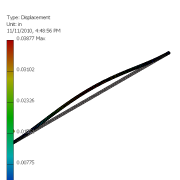
# Autodesk Inventor part: Aluminum Extrusion
Saved by Autodesk Inventor 2011 (Build 150239000, 239)
## iProperties
Created: 2010-11-11
Part Number: Aluminum Extrusion
Document SubType Name: Modeling
Designer: dfranz
Density: 2.71 g/cm^3
Material: Aluminum-6061
Mass: 2596.26 g
Surface Area: 10719.4 cm^2
Volume: 958.031 cm^3
Author: dfranz
Autodesk Inventor part; units mm, degrees
ref_plane "YZ Plane" through (0, 0, 0) normal (1, 0, 0) x (0, 1, 0)
ref_plane "XZ Plane" through (0, 0, 0) normal (0, 1, 0) x (-1, 0, 0)
ref_plane "XY Plane" through (0, 0, 0) normal (0, 0, 1) x (1, 0, 0)
sketch "Sketch1" plane through (0, 0, 0) normal (0, 0, 1) x (1, 0, 0)
  line L0 (-20.9356, 21.1258) -> (-11.0931, 21.1258)
  line L1 (8.9094, 1.1233) -> (8.9094, -8.7192)
  line L2 (-11.0931, -9.3542) -> (-20.9356, -9.3542)
  line L3 (-21.5706, 10.6483) -> (-21.5706, 20.4908)
  line L4 (-12.3631, 11.9183) -> (-0.2981, 11.9183)
  line L5 (-0.2981, 11.9183) -> (-0.2981, -0.1467)
  line L6 (-0.2981, -0.1467) -> (-12.3631, -0.1467)
  line L7 (-12.3631, -0.1467) -> (-12.3631, 11.9183)
  line L8 (-11.0931, 18.9668) -> (-19.4116, 18.9668)
  line L9 (-19.4116, 18.9668) -> (-19.4116, 10.6483)
  line L10 (-19.4116, -7.1952) -> (-11.0931, -7.1952)
  line L11 (6.7504, -7.1952) -> (6.7504, 1.1233)
  line L12 (-20.0466, 10.0133) -> (-20.9356, 10.0133)
  line L13 (-20.0466, 1.7583) -> (-20.9356, 1.7583)
  line L14 (-10.4581, 19.6018) -> (-10.4581, 20.4908)
  line L15 (-2.2031, 19.6018) -> (-2.2031, 20.4908)
  line L16 (7.3854, 10.0133) -> (8.2744, 10.0133)
  line L17 (7.3854, 1.7583) -> (8.2744, 1.7583)
  line L18 (-2.2031, -7.8302) -> (-2.2031, -8.7192)
  line L19 (-10.4581, -7.8302) -> (-10.4581, -8.7192)
  line L20 (-19.4116, 18.9668) -> (-16.2366, 18.9668)
  line L21 (-16.2366, 18.9668) -> (-16.2366, 16.4268)
  line L22 (-16.8716, 15.7918) -> (-19.4116, 15.7918)
  line L23 (-19.4116, 15.7918) -> (-19.4116, 18.9668)
  line L24 (3.5754, 18.9668) -> (6.7504, 18.9668)
  line L25 (6.7504, 18.9668) -> (6.7504, 15.7918)
  line L26 (6.7504, 15.7918) -> (4.2104, 15.7918)
  line L27 (3.5754, 16.4268) -> (3.5754, 18.9668)
  line L28 (6.7504, -7.1952) -> (3.5754, -7.1952)
  line L29 (3.5754, -7.1952) -> (3.5754, -4.6552)
  line L30 (4.2104, -4.0202) -> (6.7504, -4.0202)
  line L31 (6.7504, -4.0202) -> (6.7504, -7.1952)
  line L32 (-19.4116, -7.1952) -> (-16.2366, -7.1952)
  line L33 (-16.2366, -7.1952) -> (-16.2366, -4.0202)
  line L34 (-16.2366, -4.0202) -> (-19.4116, -4.0202)
  line L35 (-19.4116, -4.0202) -> (-19.4116, -7.1952)
  line L36 (-20.1736, 20.3638) -> (-17.6336, 20.3638)
  line L37 (-16.9986, 19.7288) -> (-16.9986, 17.1888)
  line L38 (-17.6336, 16.5538) -> (-20.1736, 16.5538)
  line L39 (-20.8086, 17.1888) -> (-20.8086, 19.7288)
  line L40 (7.5124, -8.5922) -> (4.9724, -8.5922)
  line L41 (4.3374, -7.9572) -> (4.3374, -5.4172)
  line L42 (4.9724, -4.7822) -> (7.5124, -4.7822)
  line L43 (8.1474, -5.4172) -> (8.1474, -7.9572)
  line L44 (7.5124, 20.3638) -> (4.9724, 20.3638)
  line L45 (4.3374, 19.7288) -> (4.3374, 17.1888)
  line L46 (4.9724, 16.5538) -> (7.5124, 16.5538)
  line L47 (8.1474, 17.1888) -> (8.1474, 19.7288)
  line L48 (-20.1736, -8.5922) -> (-17.6336, -8.5922)
  line L49 (-16.9986, -7.9572) -> (-16.9986, -5.4172)
  line L50 (-17.6336, -4.7822) -> (-20.1736, -4.7822)
  line L51 (-20.8086, -5.4172) -> (-20.8086, -7.9572)
  circle A0 centre (-6.884, 6.0643) radius 3.4925
  line L52 (-10.9252, 9.6564) -> (-10.4762, 10.1054)
  line L53 (-9.5781, 10.1054) -> (-2.8429, 3.3702)
  line L54 (-2.8429, 2.4722) -> (-3.2919, 2.0231)
  line L55 (-4.19, 2.0231) -> (-10.9252, 8.7583)
  line L56 (-10.4762, 2.0231) -> (-10.9252, 2.4722)
  line L57 (-10.9252, 3.3702) -> (-4.19, 10.1054)
  line L58 (-3.2919, 10.1054) -> (-2.8429, 9.6564)
  line L59 (-2.8429, 8.7583) -> (-9.5781, 2.0231)
  line L60 (-18.0326, 15.7918) -> (-12.3631, 10.1222)
  line L61 (-16.2366, 17.5878) -> (-10.567, 11.9183)
  line L62 (-2.0941, 11.9183) -> (3.5754, 17.5878)
  line L63 (-0.2981, 10.1222) -> (5.3715, 15.7918)
  line L64 (-16.2366, -5.8163) -> (-10.567, -0.1467)
  line L65 (-18.0326, -4.0202) -> (-12.3631, 1.6493)
  line L66 (3.5754, -5.8163) -> (-2.0941, -0.1467)
  line L67 (5.3715, -4.0202) -> (-0.2981, 1.6493)
  arc A1 (-20.9356, 21.1258) -> (-21.5706, 20.4908) centre (-20.9356, 20.4908) ccw
  arc A2 (-20.1736, 20.3638) -> (-20.8086, 19.7288) centre (-20.1736, 19.7288) ccw
  arc A3 (-16.9986, 19.7288) -> (-17.6336, 20.3638) centre (-17.6336, 19.7288) ccw
  arc A4 (-17.6336, 16.5538) -> (-16.9986, 17.1888) centre (-17.6336, 17.1888) ccw
  arc A5 (-20.8086, 17.1888) -> (-20.1736, 16.5538) centre (-20.1736, 17.1888) ccw
  arc A6 (-16.8716, 15.7918) -> (-16.2366, 16.4268) centre (-16.8716, 16.4268) ccw
  arc A7 (3.5754, 16.4268) -> (4.2104, 15.7918) centre (4.2104, 16.4268) ccw
  arc A8 (4.3374, 17.1888) -> (4.9724, 16.5538) centre (4.9724, 17.1888) ccw
  arc A9 (7.5124, 16.5538) -> (8.1474, 17.1888) centre (7.5124, 17.1888) ccw
  arc A10 (8.1474, 19.7288) -> (7.5124, 20.3638) centre (7.5124, 19.7288) ccw
  arc A11 (4.9724, 20.3638) -> (4.3374, 19.7288) centre (4.9724, 19.7288) ccw
  arc A12 (8.9094, 20.4908) -> (8.2744, 21.1258) centre (8.2744, 20.4908) ccw
  arc A13 (8.2744, -9.3542) -> (8.9094, -8.7192) centre (8.2744, -8.7192) ccw
  arc A14 (7.5124, -8.5922) -> (8.1474, -7.9572) centre (7.5124, -7.9572) ccw
  arc A15 (8.1474, -5.4172) -> (7.5124, -4.7822) centre (7.5124, -5.4172) ccw
  arc A16 (4.9724, -4.7822) -> (4.3374, -5.4172) centre (4.9724, -5.4172) ccw
  arc A17 (4.3374, -7.9572) -> (4.9724, -8.5922) centre (4.9724, -7.9572) ccw
  arc A18 (4.2104, -4.0202) -> (3.5754, -4.6552) centre (4.2104, -4.6552) ccw
  arc A19 (-21.5706, -8.7192) -> (-20.9356, -9.3542) centre (-20.9356, -8.7192) ccw
  arc A20 (-20.8086, -7.9572) -> (-20.1736, -8.5922) centre (-20.1736, -7.9572) ccw
  arc A21 (-17.6336, -8.5922) -> (-16.9986, -7.9572) centre (-17.6336, -7.9572) ccw
  arc A22 (-16.9986, -5.4172) -> (-17.6336, -4.7822) centre (-17.6336, -5.4172) ccw
  arc A23 (-20.1736, -4.7822) -> (-20.8086, -5.4172) centre (-20.1736, -5.4172) ccw
  arc A24 (-20.0466, 10.0133) -> (-19.4116, 10.6483) centre (-20.0466, 10.6483) ccw
  arc A25 (-21.5706, 10.6483) -> (-20.9356, 10.0133) centre (-20.9356, 10.6483) ccw
  line L68 (-21.5706, -8.7192) -> (-21.5706, 1.1233)
  line L69 (-19.4116, 1.1233) -> (-19.4116, -4.0202)
  arc A26 (-20.9356, 1.7583) -> (-21.5706, 1.1233) centre (-20.9356, 1.1233) ccw
  arc A27 (-19.4116, 1.1233) -> (-20.0466, 1.7583) centre (-20.0466, 1.1233) ccw
  arc A28 (-10.4581, -7.8302) -> (-11.0931, -7.1952) centre (-11.0931, -7.8302) ccw
  arc A29 (-11.0931, -9.3542) -> (-10.4581, -8.7192) centre (-11.0931, -8.7192) ccw
  arc A30 (8.9094, 1.1233) -> (8.2744, 1.7583) centre (8.2744, 1.1233) ccw
  arc A31 (7.3854, 1.7583) -> (6.7504, 1.1233) centre (7.3854, 1.1233) ccw
  arc A32 (-11.0931, 18.9668) -> (-10.4581, 19.6018) centre (-11.0931, 19.6018) ccw
  arc A33 (-10.4581, 20.4908) -> (-11.0931, 21.1258) centre (-11.0931, 20.4908) ccw
  line L70 (8.2744, 21.1258) -> (-1.5681, 21.1258)
  line L71 (8.9094, 20.4908) -> (8.9094, 10.6483)
  line L72 (6.7504, 10.6483) -> (6.7504, 15.7918)
  line L73 (3.5754, 18.9668) -> (-1.5681, 18.9668)
  line L74 (3.5754, -7.1952) -> (-1.5681, -7.1952)
  line L75 (8.2744, -9.3542) -> (-1.5681, -9.3542)
  arc A34 (-1.5681, -7.1952) -> (-2.2031, -7.8302) centre (-1.5681, -7.8302) ccw
  arc A35 (-2.2031, -8.7192) -> (-1.5681, -9.3542) centre (-1.5681, -8.7192) ccw
  arc A36 (8.2744, 10.0133) -> (8.9094, 10.6483) centre (8.2744, 10.6483) ccw
  arc A37 (6.7504, 10.6483) -> (7.3854, 10.0133) centre (7.3854, 10.6483) ccw
  arc A38 (-2.2031, 19.6018) -> (-1.5681, 18.9668) centre (-1.5681, 19.6018) ccw
  arc A39 (-1.5681, 21.1258) -> (-2.2031, 20.4908) centre (-1.5681, 20.4908) ccw
  arc A40 (-4.19, 2.0231) -> (-3.2919, 2.0231) centre (-3.741, 2.4722) ccw
  arc A41 (-2.8429, 2.4722) -> (-2.8429, 3.3702) centre (-3.2919, 2.9212) ccw
  arc A42 (-2.8429, 8.7583) -> (-2.8429, 9.6564) centre (-3.2919, 9.2073) ccw
  arc A43 (-3.2919, 10.1054) -> (-4.19, 10.1054) centre (-3.741, 9.6564) ccw
  arc A44 (-10.9252, 3.3702) -> (-10.9252, 2.4722) centre (-10.4762, 2.9212) ccw
  arc A45 (-10.4762, 2.0231) -> (-9.5781, 2.0231) centre (-10.0271, 2.4722) ccw
  arc A46 (-10.9252, 9.6564) -> (-10.9252, 8.7583) centre (-10.4762, 9.2073) ccw
  arc A47 (-9.5781, 10.1054) -> (-10.4762, 10.1054) centre (-10.0271, 9.6564) ccw
  arc A48 (-6.249, -0.1467) -> (-7.519, -0.1467) centre (-6.884, -0.1467) ccw
  arc A49 (-12.3631, 5.4293) -> (-12.3631, 6.6993) centre (-12.3631, 6.0643) ccw
  arc A50 (-7.519, 11.9183) -> (-6.249, 11.9183) centre (-6.884, 11.9183) ccw
  arc A51 (-0.2981, 6.6993) -> (-0.2981, 5.4293) centre (-0.2981, 6.0643) ccw
  line L76 (-16.9986, 18.9668) -> (-16.9986, 17.1888)
  line L77 (-17.6336, 16.5538) -> (-19.4116, 16.5538)
  line L78 (-16.9986, 18.9668) -> (-16.9986, 19.7288)
  line L79 (-17.6336, 20.3638) -> (-20.1736, 20.3638)
  line L80 (-20.8086, 19.7288) -> (-20.8086, 17.1888)
  line L81 (-19.4116, 16.5538) -> (-19.4116, 15.7918)
  line L82 (-16.2366, 18.9668) -> (-16.9986, 18.9668)
  arc A52 (-17.6336, 16.5538) -> (-16.9986, 17.1888) centre (-17.6336, 17.1888) ccw
  line L83 (4.3374, 18.9668) -> (4.3374, 17.1888)
  line L84 (4.9724, 16.5538) -> (6.7504, 16.5538)
  line L85 (6.7504, 16.5538) -> (7.5124, 16.5538)
  line L86 (8.1474, 17.1888) -> (8.1474, 19.7288)
  line L87 (7.5124, 20.3638) -> (4.9724, 20.3638)
  line L88 (4.3374, 19.7288) -> (4.3374, 18.9668)
  line L89 (6.7504, -4.7822) -> (4.9724, -4.7822)
  line L90 (4.3374, -5.4172) -> (4.3374, -7.1952)
  line L91 (4.3374, -7.1952) -> (4.3374, -7.9572)
  line L92 (4.9724, -8.5922) -> (7.5124, -8.5922)
  line L93 (8.1474, -7.9572) -> (8.1474, -5.4172)
  line L94 (7.5124, -4.7822) -> (6.7504, -4.7822)
  line L95 (6.7504, -4.7822) -> (4.9724, -4.7822)
  line L96 (-16.9986, -7.1952) -> (-16.9986, -5.4172)
  line L97 (-17.6336, -4.7822) -> (-19.4116, -4.7822)
  line L98 (-19.4116, -4.7822) -> (-20.1736, -4.7822)
  line L99 (-20.8086, -5.4172) -> (-20.8086, -7.9572)
  line L100 (-20.1736, -8.5922) -> (-17.6336, -8.5922)
  line L101 (-16.9986, -7.9572) -> (-16.9986, -7.1952)
  point P0 (0, 0)
  point P1 (0, 0)
  point P2 (-21.5706, 21.1258)
  point P3 (8.9094, -9.3542)
  point P4 (8.9094, 21.1258)
  point P5 (-19.4116, 1.7583)
  point P6 (-21.5706, 1.7583)
  point P7 (-2.2031, 18.9668)
  point P8 (-2.2031, 21.1258)
  point P9 (6.7504, 10.0133)
  point P10 (8.9094, 10.0133)
  point P11 (-2.2031, -7.1952)
  point P12 (-2.2031, -9.3542)
  point P13 (-16.2366, 15.7918)
  point P14 (3.5754, 15.7918)
  point P15 (3.5754, -4.0202)
  point P16 (-16.9986, 16.5538)
  point P17 (-16.9986, 20.3638)
  point P18 (-20.8086, 16.5538)
  point P19 (8.1474, -8.5922)
  point P20 (4.3374, -8.5922)
  point P21 (8.1474, -4.7822)
  point P22 (-11.3742, 9.2073)
  point P23 (-2.3939, 2.9212)
  point P24 (-10.0271, 10.5544)
  point P25 (-10.0271, 1.5741)
  point P26 (-3.741, 10.5544)
  point P27 (-11.3742, 2.9212)
  dimension "d0" = 30.48
  dimension "d1" = 30.48
  dimension "d2" = 12.065
  dimension "d3" = 12.065
  dimension "d4" = 9.2075
  dimension "d5" = 9.2075
  dimension "d6" = 9.2075
  dimension "d7" = 2.159
  dimension "d8" = 8.255
  dimension "d9" = 11.1125
  dimension "d10" = 8.255
  dimension "d11" = 11.1125
  dimension "d12" = 3.175
  dimension "d13" = 3.175
  dimension "d14" = 3.175
  dimension "d15" = 3.175
  dimension "d16" = 3.81
  dimension "d17" = 3.81
  dimension "d18" = 0.762
  dimension "d19" = 0.762
  dimension "d20" = 0.762
  dimension "d21" = 3.81
  dimension "d22" = 3.81
  dimension "d23" = 0.762
  dimension "d24" = 0.762
  dimension "d25" = 6.985
  dimension "d26" = 10.795
  dimension "d27" = 1.905
  dimension "d28" = 1.905
  dimension "d29" = 10.795
  dimension "d30" = 5.3975
  dimension "d31" = 5.3975
  dimension "d32" = 0.9525
  dimension "d33" = 0.9525
  dimension "d34" = 5.3975
  dimension "d35" = 0.9525
  dimension "d36" = 2.54
  dimension "d37" = 1.27
  dimension "d38" = 2.54
  dimension "d39" = 1.27
  dimension "d40" = 2.54
  dimension "d41" = 0
  dimension "d42" = 1.27
  dimension "d43" = 2.54
  dimension "d44" = 1.27
  dimension "d45" = 0.635
  dimension "d46" = 0.635
  dimension "d47" = 0.635
  dimension "d48" = 0.635
  dimension "d49" = 0.635
  dimension "d50" = 0
  dimension "d51" = 0
  dimension "d52" = 0.635
  dimension "d53" = 0
  dimension "d54" = 0.635
  dimension "d55" = 0
  dimension "d56" = 0
  dimension "d57" = 0
  dimension "d58" = 0.635
  dimension "d59" = 0
  dimension "d60" = 0
  dimension "d63" = 30.48
  constraints: 204 end point, 120 tangent, 110 point on line, 104 point on circle, 53 centre point, 43 equal radius, 35 parallel, 34 perpendicular, 14 collinear, 10 horizontal, 3 other
  measures "d0" distance of point (-21.571, 21.126) point (8.909, 21.126)
  measures "d1" distance of point (8.909, 21.126) point (8.909, -9.354)
  measures "d2" distance of L4.start L5.start
  measures "d3" distance of L5.start L5.end
  measures "d4" distance between parallel lines of L2 L6
  measures "d5" distance between parallel lines of L0 L4
  measures "d6" distance between parallel lines of L3 L7
  measures "d7" distance between parallel lines of L0 L8
  measures "d8" distance between parallel lines of L12 L13
  measures "d9" distance between parallel lines of L0 L12
  measures "d10" distance between parallel lines of L15 L14
  measures "d11" distance between parallel lines of L1 L15
  measures "d12" distance of L21.start point (-16.237, 15.792)
  measures "d13" distance of point (-16.237, 15.792) L23.start
  measures "d14" distance of L25.end point (3.575, 15.792)
  measures "d15" distance of L28.end point (3.575, -4.02)
  measures "d16" distance of point (-16.999, 20.364) point (-16.999, 16.554)
  measures "d17" distance of point (-16.999, 16.554) point (-20.809, 16.554)
  measures "d18" distance between parallel lines of L0 L36
  measures "d19" distance between parallel lines of L3 L39
  measures "d20" distance between parallel lines of L22 L38
  measures "d21" distance of point (8.147, -4.782) point (8.147, -8.592)
  measures "d22" distance of point (8.147, -8.592) point (4.337, -8.592)
  measures "d23" distance between parallel lines of L2 L40
  measures "d24" distance between parallel lines of L1 L43
  measures "d25" diameter of A0
  measures "d26" distance of point (-10.027, 10.554) point (-2.394, 2.921)
  measures "d27" distance of point (-11.374, 9.207) point (-10.027, 10.554)
  measures "d28" distance of point (-10.027, 1.574) point (-11.374, 2.921)
  measures "d29" distance of point (-11.374, 2.921) point (-3.741, 10.554)
  measures "d30" distance from line of L52 A0.centre
  measures "d31" distance from line of L54 A0.centre
  measures "d32" distance from line of L57 A0.centre
  measures "d33" distance from line of A0.centre L59
  measures "d34" distance from line of L58 A0.centre
  measures "d35" distance from line of A0.centre L53
  measures "d36" distance between parallel lines of L61 L60
  measures "d37" distance from line of point (-16.237, 15.792) L60
  measures "d38" distance between parallel lines of L62 L63
  measures "d39" distance from line of L5.start L63
  measures "d40" distance between parallel lines of L65 L64
  measures "d41" distance between parallel lines of L21 L33
  measures "d42" distance from line of L33.end L64
  measures "d43" distance between parallel lines of L66 L67
  measures "d44" distance from line of point (3.575, -4.02) L67
  measures "d45" radius of A1
  measures "d46" radius of A24
  measures "d47" radius of A26
  measures "d48" radius of A34
  measures "d49" radius of A48
  measures "d50" distance from line of L6 A48.centre
  measures "d51" horizontal distance of A0.centre A48.centre
  measures "d52" radius of A49
  measures "d53" vertical distance of A0.centre A49.centre
  measures "d54" radius of A50
  measures "d55" distance from line of L4 A50.centre
  measures "d56" horizontal distance of A0.centre A50.centre
  measures "d57" distance from line of L7 A49.centre
  measures "d58" radius of A51
  measures "d59" distance from line of L5 A51.centre
  measures "d60" vertical distance of A0.centre A51.centre
  measures "d63" distance between parallel lines of L71 L3
extrude "Extrusion1" add sketch "Sketch1" along normal blind 3048 contours L0 A33 L14 A32 L8 L37 A3 L36 A2 L39 A5 L38 L9 A24 L12 A25 L3 A1 | L21 A6 L22 L9 L38 A4 L37 L8 | L61 L4 L7 L60 L22 A6 L21 | L4 A50 L5 A51 L6 A48 L7 A49 | L62 L27 A7 L26 L63 L5 L4 | L27 L24 L45 A8 L46 L25 L26 A7 | L7 L6 L64 L33 L34 L65 | L73 A38 L15 A39 L70 A12 L71 A36 L16 A37 L72 L25 L46 A9 L47 A10 L44 A11 L45 L24 | L34 L33 L10 L49 A22 L50 L35 | L35 L50 A23 L51 A20 L48 A21 L49 L10 A28 L19 A29 L2 A19 L68 A26 L13 A27 L69 | L67 L30 A18 L29 L66 L6 L5 | L30 L11 L42 A16 L41 L28 L29 A18 | L11 A31 L17 A30 L1 A13 L75 A35 L18 A34 L74 L28 L41 A17 L40 A14 L43 A15 L42
body "Solid1"
